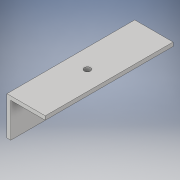
# Autodesk Inventor part: 30x30L
Saved by Autodesk Inventor 2019 (Build 230136000, 136)
## iProperties
Created: 2022-08-27
Part Number: 30x30L
Material: Generic
Document SubType Name: Modeling
Designer: laca
Density: 1 g/cm^3
Appearance: Default
Author: laca
Autodesk Inventor part; units mm, degrees
ref_plane "YZ Plane" through (0, 0, 0) normal (1, 0, 0) x (0, 1, 0)
ref_plane "XZ Plane" through (0, 0, 0) normal (0, 1, 0) x (-1, 0, 0)
ref_plane "XY Plane" through (0, 0, 0) normal (0, 0, 1) x (1, 0, 0)
sketch "Sketch1" plane through (0, 0, 0) normal (0, 0, 1) x (1, 0, 0)
  line L0 (-49.4183, -0.4981) -> (-49.4183, 29.5019)
  line L1 (-49.4183, 29.5019) -> (-19.4183, 29.5019)
  line L2 (-19.4183, 29.5019) -> (-19.4183, 26.5019)
  line L3 (-19.4183, 26.5019) -> (-46.4183, 26.5019)
  line L4 (-46.4183, 26.5019) -> (-46.4183, -0.4981)
  line L5 (-49.4183, -0.4981) -> (-46.4183, -0.4981)
  point P0 (0, 0)
  dimension "d0" = 30
  dimension "d1" = 30
  dimension "d2" = 27
  dimension "d3" = 3
  constraints: 12 end point, 3 perpendicular, 2 vertical, 1 horizontal
  measures "d0" distance of L0.end L1.end
  measures "d1" distance of L0.start L0.end
  measures "d2" distance of L2.end L3.end
  measures "d3" distance between parallel lines of L1 L3
extrude "Extrusion1" add sketch "Sketch1" along normal blind 100
sketch "Sketch2" plane through (-49.4183, 29.5019, 0) normal (0, 1, 0) x (1, 0, 0)
  circle A0 centre (15, -52.0193) radius 2.4561
  line L0 (0, 0) -> (0, -100) projected
  point P0 (49.4183, 0)
  dimension "d6" = 15
  constraints: 1 centre point
  measures "d6" distance from line of L0 A0.centre
extrude "Extrusion2" cut sketch "Sketch2" against normal through all
body "Solid1"
